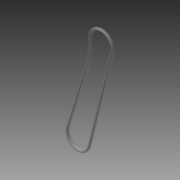
# Autodesk Inventor part: Polycord
Saved by Autodesk Inventor 2014 SP1 (Build 180222100, 222)
## iProperties
Created: 2012-03-30
Part Number: Polycord
Material: Generic
Document SubType Name: Modeling
Designer: Moses
Density: 1 g/cm^3
Mass: 13.4922 g
Surface Area: 169.981 cm^2
Volume: 13.4922 cm^3
Appearance: Polycarbonate - Clear
Author: Moses
Autodesk Inventor part; units mm, degrees
ref_plane "YZ Plane" through (0, 0, 0) normal (1, 0, 0) x (0, 1, 0)
ref_plane "XZ Plane" through (0, 0, 0) normal (0, 1, 0) x (-1, 0, 0)
sketch "Sketch1" plane through (0, 0, 0) normal (0, 0, 1) x (1, 0, 0)
  circle A0 centre (0, 0) radius 21.082 construction
  circle A1 centre (-49.6338, -201.248) radius 21.082 construction
  arc A2 (23.5513, -5.8085) -> (-24.2381, 0.9575) centre (0, 0) ccw
  arc A3 (-72.8413, -194.19) -> (-26.0825, -207.0564) centre (-49.6338, -201.248) ccw
  circle A4 centre (-34.6801, -38.1566) radius 5.715 construction
  arc A5 (-26.1748, -40.7433) -> (-25.7971, -38.5075) centre (-34.6801, -38.1566) ccw
  line L0 (-26.1748, -40.7433) -> (-72.8413, -194.19)
  line L1 (-26.0825, -207.0564) -> (23.5513, -5.8085)
  line L2 (-24.2381, 0.9575) -> (-25.7971, -38.5075)
  point P0 (0, 0)
  dimension "d0" = 11.43
  dimension "d1" = 17.78
  dimension "d2" = 42.164
  dimension "d3" = 48.514
  dimension "d4" = 42.164
  dimension "d5" = 48.514
  constraints: 6 end point, 6 point on circle, 6 tangent, 3 centre point, 3 coincident
  measures "d0" diameter of A4
  measures "d1" diameter of A5
  measures "d2" diameter of A0
  measures "d3" diameter of A2
  measures "d4" diameter of A1
  measures "d5" diameter of A3
ref_plane "Work Plane1" through (-72.8413, -194.19, 0) normal (-0.2909642, -0.956734, 0) x (0.956734, -0.2909642, 0)
sketch "Sketch2" plane through (-72.8413, -194.19, 0) normal (-0.2909642, -0.956734, 0) x (0.956734, -0.2909642, 0)
  circle A0 centre (0, 0) radius 3.175
  circle A1 centre (0, 0) radius 1.5875
  point P0 (13.1874, 0)
  dimension "d6" = 6.35
  dimension "d7" = 3.175
  constraints: 2 centre point, 2 coincident
  measures "d6" diameter of A0
  measures "d7" diameter of A1
sweep "Sweep1" add profiles "Sketch2" path "Sketch1"
body "Solid1"
